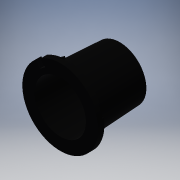
# Autodesk Inventor part: Base
Saved by Autodesk Inventor 2016 (Build 200138000, 138)
## iProperties
Created: 2015-05-26
Part Number: Base
Material: Generic
Document SubType Name: Modeling
Designer: Andy
Density: 0.619476 g/cm^3
Appearance: Default
Mass: 914 g
Surface Area: 2729.39 cm^2
Volume: 1475.44 cm^3
Author: Andy
Autodesk Inventor part; units mm, degrees
ref_plane "YZ Plane" through (0, 0, 0) normal (1, 0, 0) x (0, 1, 0)
sketch "Sketch2" plane through (0, 0, 0) normal (0, 1, 0) x (-1, 0, 0)
  circle A0 centre (0, 0) radius 119.85625
  dimension "d1" = 239.7125
  constraints: 1 centre point, 1 coincident
  measures "d1" diameter of A0
extrude "Extrusion1" add sketch "Sketch2" along normal blind 19.05
ref_plane "Work Plane1" through (0, 187.325, 0) normal (0, 1, 0) x (1, 0, 0)
sketch "Sketch3" plane through (0, 187.325, 0) normal (0, 1, 0) x (1, 0, 0)
  circle A0 centre (0, 0) radius 84.1375
  circle A1 centre (0, 0) radius 75.1375
  dimension "d5" = 168.275
  dimension "d6" = 9
  constraints: 2 centre point, 2 coincident
  measures "d5" diameter of A0
  measures "d6" radial gap between concentric circles of A0 A1
sketch "Sketch5" plane through (0, 19.05, 0) normal (0, 1, 0) x (1, 0, 0)
  circle A0 centre (0, 0) radius 119.85625
  circle A1 centre (0, 0) radius 92.85625
  circle A2 centre (0, 0) radius 83.85625
  dimension "d7" = 27
  dimension "d8" = 9
  constraints: 2 centre point, 2 coincident
  measures "d7" radial gap between concentric circles of A1 A0
  measures "d8" radial gap between concentric circles of A1 A2
loft "Loft1" add profiles "Sketch5", "Sketch3" contours A1 | A2 / A0 | A1
sketch "Sketch6" plane through (0, 187.325, 0) normal (0, 1, 0) x (1, 0, 0)
  circle A0 centre (0, 0) radius 84.1375 projected
  circle A1 centre (0, 0) radius 75.1375
  dimension "d13" = 9
  constraints: 1 centre point, 1 coincident
  measures "d13" radial gap between concentric circles of A1 A0
sketch "Sketch7" plane through (0, 0, 0) normal (0, -1, 0) x (1, 0, 0)
  circle A0 centre (0, 0) radius 119.85625
  circle A1 centre (0, 0) radius 80.9625
  dimension "d14" = 161.925
  constraints: 1 centre point, 1 coincident
  measures "d14" diameter of A1
loft "Loft2" cut profiles "Sketch6", "Sketch7" contours A1 / A1
sketch "Sketch8" plane through (0, 19.05, 0) normal (0, 1, 0) x (1, 0, 0)
  circle A0 centre (0, 0) radius 92.85625
  circle A1 centre (0, 0) radius 119.85625
  circle A2 centre (0, 0) radius 119.85625
  line L0 (-17.5, -67.140705) -> (17.5, -118.571795) construction
  line L1 (17.5, -67.140705) -> (-17.5, -118.571795) construction
  line L2 (0, -92.85625) -> (0, -104.85625)
  arc A3 (9.049411, -100.600882) -> (-9.049411, -100.600882) centre (0, -104.85625) ccw
  line L3 (17.5, -118.571795) -> (9.049411, -100.600882)
  line L4 (-17.5, -118.571795) -> (-9.049411, -100.600882)
  arc A4 (-17.5, -118.571795) -> (17.5, -118.571795) centre (0, 0) ccw
  arc A5 (98.473546, -22.480881) -> (92.880702, -39.693884) centre (99.72422, -32.402363) ccw
  line L5 (118.176276, -19.997211) -> (98.473546, -22.480881)
  line L6 (107.360681, -53.284189) -> (92.880702, -39.693884)
  arc A6 (107.360681, -53.284189) -> (118.176276, -19.997211) centre (0, 0) ccw
  arc A7 (51.810587, 86.706933) -> (66.452842, 76.068713) centre (61.632957, 84.830488) ccw
  line L7 (55.536955, 106.212839) -> (51.810587, 86.706933)
  line L8 (83.85255, 85.640356) -> (66.452842, 76.068713)
  arc A8 (83.85255, 85.640356) -> (55.536955, 106.212839) centre (0, 0) ccw
  arc A9 (-66.452842, 76.068713) -> (-51.810587, 86.706933) centre (-61.632957, 84.830488) ccw
  line L9 (-83.85255, 85.640356) -> (-66.452842, 76.068713)
  line L10 (-55.536955, 106.212839) -> (-51.810587, 86.706933)
  arc A10 (-55.536955, 106.212839) -> (-83.85255, 85.640356) centre (0, 0) ccw
  arc A11 (-92.880702, -39.693884) -> (-98.473546, -22.480881) centre (-99.72422, -32.402363) ccw
  line L11 (-107.360681, -53.284189) -> (-92.880702, -39.693884)
  line L12 (-118.176276, -19.997211) -> (-98.473546, -22.480881)
  arc A12 (-118.176276, -19.997211) -> (-107.360681, -53.284189) centre (0, 0) ccw
  dimension "d19" = 35
  dimension "d20" = 12
  dimension "d21" = 20
  dimension "d24" = 360
  constraints: 26 end point, 20 point on circle, 10 centre point, 2 midpoint, 2 tangent, 1 coincident, 1 vertical, 1 vertical alignment, 54 other
  measures "d19" distance of L0.end L1.end
  measures "d20" distance of L2.start L2.end
  measures "d21" diameter of A3
extrude "Extrusion2" cut sketch "Sketch8" against normal blind 4 contours L8 A7 L7 A1 | A1 L6 A5 L5 | L10 A9 L9 A1 | A1 L4 A3 L3 | L12 A11 L11 A1
sketch "Sketch9" plane through (0, 19.05, 0) normal (0, 1, 0) x (1, 0, 0)
  circle A0 centre (0, 0) radius 119.85625
  line L0 (-61.550549, -103.431381) -> (-79.348923, -90.500105)
  line L1 (-61.550549, -103.431381) -> (-48.031488, -84.82399)
  line L2 (-48.031488, -84.82399) -> (-65.829862, -71.892714)
  line L3 (-65.829862, -71.892714) -> (-79.348923, -90.500105)
  dimension "d28" = 22
  dimension "d29" = 23
  constraints: 8 end point, 1 perpendicular
  measures "d28" distance of L0.start L0.end
  measures "d29" distance of L0.start L1.end
extrude "Extrusion3" cut sketch "Sketch9" against normal through all contours L3 L2 L1 A0 | A0 L0 L3 | L1 L0 A0 picked at (-61.437029, -84.560815)
ref_plane "Work Plane2" through (0, 182.325, 0) normal (0, 1, 0) x (1, 0, 0)
ref_plane "Work Plane3" through (0, 172.325, 0) normal (0, 1, 0) x (1, 0, 0)
sketch "Sketch11" plane through (0, 182.325, 0) normal (0, 1, 0) x (1, 0, 0)
  circle A0 centre (0, 0) radius 75.1375
  circle A1 centre (0, 0) radius 80.9625
  circle A2 centre (0, 0) radius 75.1375
  circle A3 centre (0, 0) radius 75.292978
  circle A4 centre (0, 0) radius 84.396563
  circle A5 centre (0, 0) radius 75.1375
  circle A6 centre (0, 0) radius 53.1375
  dimension "d39" = 22
  constraints: 3 centre point, 3 coincident, 1 concentric
  measures "d39" radial gap between concentric circles of A6 A0
sketch "Sketch12" plane through (0, 172.325, 0) normal (0, 1, 0) x (1, 0, 0)
  circle A0 centre (0, 0) radius 75.603935
  circle A1 centre (0, 0) radius 84.914688
  circle A2 centre (0, 0) radius 75.603935
  constraints: 1 centre point, 1 coincident, 1 concentric
sketch "Sketch11 outline for Loft3" plane through (0, 182.325, 0) normal (0, 1, 0) x (1, 0, 0)
  circle A0 centre (0, 0) radius 75.1375
loft "Loft3" add profiles "Sketch11 outline for Loft3", "Sketch12" contours all / A0
extrude "Extrusion4" cut sketch "Sketch11" against normal through all contours A6
sketch "Sketch13" plane through (0, 182.325, 0) normal (0, 1, 0) x (1, 0, 0)
  circle A0 centre (0, 0) radius 75.1375
  line L0 (-48.031488, -84.82399) -> (-61.253225, -103.022149)
  line L1 (-79.051599, -90.090873) -> (-65.829862, -71.892714)
  line L2 (-65.829862, -71.892714) -> (-48.031488, -84.82399)
  line L3 (-56.930675, -78.358352) -> (44.164714, 60.787514)
  line L4 (-96.325661, 10.124235) -> (74.725889, -7.854007)
  line L5 (-39.394986, 88.482587) -> (30.561175, -68.641522)
  line L6 (56.930675, 78.358352) -> (-44.164714, -60.787514)
  line L7 (96.325661, -10.124235) -> (-74.725889, 7.854007)
  line L8 (39.394986, -88.482587) -> (-30.561175, 68.641522)
  line L9 (-39.394986, 88.482587) -> (56.930675, 78.358352)
  line L10 (8.767845, 83.42047) -> (0, 0)
  line L11 (22.613739, 71.65377) -> (18.526572, 32.766978)
  line L12 (18.526572, 32.766978) -> (-11.309084, 35.902832)
  line L13 (-11.309084, 35.902832) -> (-7.221918, 74.789624)
  line L14 (-0.990883, 134.073961) -> (18.526572, 32.766978) construction
  line L15 (28.844774, 130.938107) -> (-11.309084, 35.902832) construction
  line L16 (-7.221918, 74.789624) -> (22.613739, 71.65377)
  dimension "d48" = 360
  dimension "d50" = 30
  constraints: 28 end point, 4 midpoint, 3 point on circle, 2 parallel, 1 perpendicular, 19 other
  measures "d50" distance of L14.start L15.start
extrude "Extrusion5" cut sketch "Sketch13" against normal through all contours L11 L12 L10 L16 | L10 L12 L13 L16
sketch "Sketch14" plane through (0, 182.325, 0) normal (0, 1, 0) x (0.9945219, 0, 0.1045285)
  arc A0 (-15, 73.625022) -> (15, 73.625022) centre (0, 0) ccw
  line L0 (-57.954404, -78.379973) -> (-38.901846, -89.379973)
  circle A1 centre (0, 0) radius 75.603935
  line L1 (-48.428125, -83.879973) -> (0, 0)
  line L2 (48.428125, -83.879973) -> (0, 0)
  line L3 (96.85625, 0) -> (0, 0)
  line L4 (48.428125, 83.879973) -> (0, 0)
  line L5 (-48.428125, 83.879973) -> (0, 0)
  line L6 (-96.85625, 0) -> (0, 0)
  line L7 (0, -75.1375) -> (0, -67.1375)
  arc A2 (-15, 50.976405) -> (15, 50.976405) centre (0, 0) ccw
  arc A3 (-26.56875, -46.018425) -> (26.56875, -46.018425) centre (0, -39.865619) ccw
  dimension "d55" = 360
  constraints: 14 end point, 6 point on circle, 2 point on line, 1 centre point, 1 midpoint, 1 vertical, 1 vertical alignment, 20 other
extrude "Extrusion6" cut sketch "Sketch14" against normal through all contours A2 A3
sketch "Sketch15" plane through (-48.031488, 0, 84.82399) normal (-0.5877853, 0, 0.809017) x (0.809017, 0, 0.5877853)
  line L0 (0, 0) -> (-22, 0) projected
  line L1 (0, 19.05) -> (0, 0) projected
  line L2 (-22, 19.05) -> (0, 19.05) projected
  line L3 (-22, 19.05) -> (-22, 0) projected
  line L4 (-22, 0) -> (0, 0)
  line L5 (0, 0) -> (0, 62)
  line L6 (0, 62) -> (-22, 62)
  line L7 (-22, 62) -> (-22, 0)
  point P0 (-11, 0)
  dimension "d60" = 62
  constraints: 8 end point, 2 parallel, 1 horizontal, 1 perpendicular
  measures "d60" distance of L5.end L4.end
extrude "Extrusion7" add sketch "Sketch15" against normal up to next contours L2 L7 L6 L5
sketch "Sketch16" plane through (-48.031488, 19.05, 84.82399) normal (-0.5877853, 0, 0.809017) x (0.809017, 0, 0.5877853)
  line L0 (0, 42.95) -> (-22, 42.95) projected
  line L1 (-11, -19.05) -> (-11, -3.05) construction
  circle A0 centre (-11, -3.05) radius 5
  line L2 (-11, 42.95) -> (-11, 20.45) construction
  circle A1 centre (-11, 20.45) radius 5
  dimension "d63" = 16
  dimension "d64" = 10
  dimension "d65" = 22.5
  dimension "d66" = 10
  constraints: 4 end point, 2 centre point, 2 coincident, 2 vertical, 1 midpoint
  measures "d63" distance of L1.start L1.end
  measures "d64" diameter of A0
  measures "d65" distance of L2.start L2.end
  measures "d66" diameter of A1
extrude "Extrusion8" cut sketch "Sketch16" against normal blind 20
body "Solid1"
